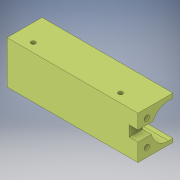
# Autodesk Inventor part: bATTERYrAILS
Saved by Autodesk Inventor 2019 (Build 230136000, 136)
## iProperties
Created: 2019-09-28
Part Number: bATTERYrAILS
Material: Generic
Document SubType Name: Modeling
Designer: james
Density: 1 g/cm^3
Appearance: Default(1)
Author: james
Autodesk Inventor part; units mm, degrees
ref_plane "YZ Plane" through (0, 0, 0) normal (1, 0, 0) x (0, 1, 0)
ref_plane "XZ Plane" through (0, 0, 0) normal (0, 1, 0) x (-1, 0, 0)
ref_plane "XY Plane" through (0, 0, 0) normal (0, 0, 1) x (1, 0, 0)
sketch "Sketch1" plane through (0, 0, 0) normal (1, 0, 0) x (0, 1, 0)
  line L0 (0, 0) -> (31.115, 0)
  line L1 (31.115, 0) -> (31.115, 25.4)
  line L2 (31.115, 25.4) -> (0, 25.4)
  line L3 (0, 25.4) -> (0, 0)
  dimension "d0" = 25.4
  dimension "d1" = 31.115
  constraints: 8 end point, 2 parallel, 1 horizontal, 1 perpendicular
  measures "d0" distance of L2.end L0.start
  measures "d1" distance of L1.end L2.end
extrude "Extrusion1" add sketch "Sketch1" along normal blind 95.25
sketch "Sketch2" plane through (95.25, 0, 0) normal (1, 0, 0) x (0, 0, -1)
  arc A0 (-3.175, 27.94) -> (-3.175, 2.54) centre (-3.175, 15.24) ccw
  line L0 (0, 0) -> (0, 31.115) projected
  line L1 (-25.4, 0) -> (0, 0) projected
  line L2 (-3.175, 27.94) -> (0, 27.94)
  line L3 (-3.175, 2.54) -> (0, 2.54)
  dimension "d4" = 3.175
  dimension "d5" = 15.24
  dimension "d6" = 25.4
  constraints: 4 end point, 2 point on circle, 2 point on line, 2 tangent, 1 centre point, 1 horizontal, 1 perpendicular
  measures "d4" distance from line of L0 A0.centre
  measures "d5" distance from line of L1 A0.centre
  measures "d6" diameter of A0
extrude "Extrusion2" cut sketch "Sketch2" against normal blind 88.9
sketch "Sketch3" plane through (0, 31.115, 25.4) normal (0, 1, 0) x (1, 0, 0)
  line L0 (0, 25.4) -> (0, 0) projected
  line L1 (95.25, 25.4) -> (95.25, 0) projected
  line L2 (0, 0) -> (95.25, 0) projected
  point P0 (12.7, 6.35)
  point P1 (76.2, 6.35)
  dimension "d9" = 0
  dimension "d10" = 12.7
  dimension "d12" = 6.35
  dimension "d35" = 76.2
  measures "d9" vertical distance of point (12.7, 6.35) point (76.2, 6.35)
  measures "d10" distance from line of L0 point (12.7, 6.35)
  measures "d12" distance from line of L2 point (76.2, 6.35)
  measures "d35" distance from line of L0 point (76.2, 6.35)
hole "Hole1" at (12.7, 31.115, 19.05) at (76.2, 31.115, 19.05) direction (0, -1, 0) diameter 3.175 end through all
sketch "Sketch4" plane through (95.25, 0, 0) normal (1, 0, 0) x (0, 0, -1)
  line L0 (-10.782, 20.574) -> (-30.1642, 20.574)
  line L1 (-30.1642, 20.574) -> (-30.1642, 12.954)
  line L2 (-30.1642, 12.954) -> (-10.782, 12.954)
  line L3 (-10.782, 12.954) -> (-10.782, 20.574)
  line L4 (-25.4, 0) -> (0, 0) projected
  dimension "d20" = 7.62
  dimension "d21" = 12.954
  constraints: 8 end point, 2 parallel, 1 horizontal, 1 perpendicular
  measures "d20" distance of L0.end L1.end
  measures "d21" distance between parallel lines of L4 L2
extrude "Extrusion3" cut sketch "Sketch4" against normal blind 6.35
sketch "Sketch5" plane through (95.25, 0, 0) normal (1, 0, 0) x (0, 0, -1)
  line L0 (-25.4, 12.954) -> (-25.4, 0) projected
  line L1 (-25.4, 0) -> (0, 0) projected
  line L2 (-25.4, 31.115) -> (-25.4, 20.574) projected
  line L3 (0, 31.115) -> (-25.4, 31.115) projected
  point P0 (-19.05, 24.765)
  point P1 (-19.05, 6.35)
  dimension "d24" = 6.35
  dimension "d25" = 6.35
  dimension "d26" = 6.35
  dimension "d27" = 6.35
  measures "d24" distance from line of L0 point (-19.05, 6.35)
  measures "d25" distance from line of L1 point (-19.05, 6.35)
  measures "d26" distance from line of L2 point (-19.05, 24.765)
  measures "d27" distance from line of L3 point (-19.05, 24.765)
hole "Hole2" at (95.25, 24.765, 19.05) at (95.25, 6.35, 19.05) direction (-1, 0, 0) diameter 3.81 depth 12.7 tip angle 118.188
body "Solid1"
